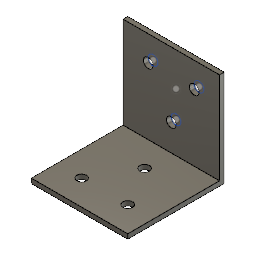
08part (Autodesk Fusion 360 design; units mm, degrees)
Autodesk Fusion 360 part; units mm, degrees
sketch "Sketch1" plane through (0, 0, 0) normal (1, 0, 0) x (0, 0, -1)
  line L0 (0, 40) -> (-2, 40)
  line L1 (-2, 40) -> (-2, 0)
  line L2 (-2, 0) -> (0, 0)
  line L3 (0, 0) -> (0, 40)
  line L4 (0, 0) -> (-40, 0)
  line L5 (-40, 0) -> (-40, 2)
  line L6 (-40, 2) -> (0, 2)
  line L7 (0, 2) -> (0, 0)
  dimension "d1" = 2
  dimension "d2" = 40
  constraint horizontal L0
  constraint vertical L1
  constraint horizontal L2
  constraint vertical L3
  constraint coincident L2.end L3.start
  constraint horizontal L4
  constraint vertical L5
  constraint horizontal L6
  constraint vertical L7
  constraint equal L3 L6
  constraint equal L0 L5
  measures "d1" distance of L0.start L0.end
  measures "d2" distance of L0.start L2.end
extrude "Extrude1" add sketch "Sketch1" along normal blind 40
sketch "Sketch2" plane through (0, 0, 0) normal (0, 0, -1) x (-1, 0, 0)
  circle A0 centre (-20, 13) radius 2
  circle A1 centre (-10.4737, 29.5) radius 2
  circle A2 centre (-29.5263, 29.5) radius 2
  point P0 (-20, 24)
  dimension "d5" = 4
  dimension "d8" = 360
  measures "d5" diameter of A0
extrude "Extrude2" cut sketch "Sketch2" against normal blind 2
ref_plane "WorkPlane1" through (0, 2, 2) normal (0, -0.707107, 0.707107) x (1, 0, 0)
mirror "Mirror1" about plane through (0, 2, 2) normal (0, -0.707107, 0.707107) of "Extrude2"
